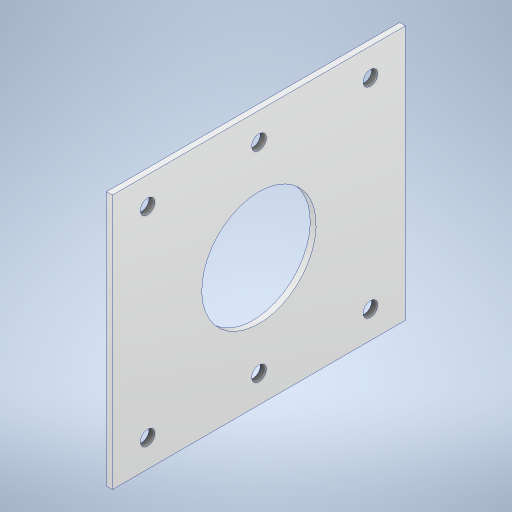
# Autodesk Inventor part: mount_plate_4x2020
Saved by Autodesk Inventor 2024 (Build 280153000, 153)
## iProperties
Created: 2025-12-15
Part Number: mount_plate_4x2020
Material: Aluminum 6061
Document SubType Name: Modeling
Designer: schar
Density: 2.7 g/cm^3
Appearance: Aluminum - Flat
Author: schar
Autodesk Inventor part; units mm, degrees
ref_plane "YZ Plane" through (0, 0, 0) normal (1, 0, 0) x (0, 1, 0)
ref_plane "XZ Plane" through (0, 0, 0) normal (0, 1, 0) x (-1, 0, 0)
ref_plane "XY Plane" through (0, 0, 0) normal (0, 0, 1) x (1, 0, 0)
sketch "Sketch1" plane through (0, 0, 0) normal (1, 0, 0) x (0, 1, 0)
  circle A0 centre (0, 0) radius 19.5
  line L0 (43.5, 50) -> (-43.5, 50)
  line L1 (-43.5, 50) -> (-43.5, -50)
  line L2 (-43.5, -50) -> (43.5, -50)
  line L3 (43.5, -50) -> (43.5, 50)
  line L4 (43.5, 50) -> (-43.5, -50) construction
  line L5 (-43.5, 50) -> (43.5, -50) construction
  line L6 (0, 0) -> (0, -38)
  line L7 (0, -38) -> (34.15, -38)
  circle A1 centre (34.15, -38) radius 2.5
  circle A2 centre (-34.15, -38) radius 2.5
  circle A3 centre (34.15, 0) radius 2.5
  circle A4 centre (-34.15, 0) radius 2.5
  circle A5 centre (34.15, 38) radius 2.5
  circle A6 centre (-34.15, 38) radius 2.5
  dimension "d0" = 39
  dimension "d1" = 87
  dimension "d2" = 100
  dimension "d3" = 38
  dimension "d4" = 34.15
  dimension "d5" = 5
  dimension "d8" = 68.3
  dimension "d11" = 38
  constraints: 16 end point, 7 centre point, 2 coincident, 2 horizontal, 2 midpoint, 2 parallel, 2 perpendicular, 2 vertical, 10 other
  measures "d0" diameter of A0
  measures "d1" distance of L2.end L1.end
  measures "d2" distance of L1.end L0.end
  measures "d3" distance of L6.start L6.end
  measures "d4" distance of L6.end L7.end
  measures "d5" diameter of A1
  measures "d8" distance of A1.centre A2.centre
  measures "d11" distance of A1.centre A3.centre
extrude "Extrusion1" add sketch "Sketch1" along normal blind 2
body "Solid1"
